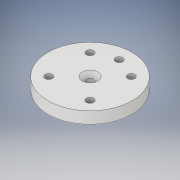
# Autodesk Inventor part: baseplate
Saved by Autodesk Inventor 2019 (Build 230136000, 136)
## iProperties
Created: 2019-05-05
Part Number: baseplate
Material: PBT Plastic
Document SubType Name: Modeling
Designer: infinity
Density: 1.31 g/cm^3
Appearance: Smooth - White
Author: infinity
Autodesk Inventor part; units mm, degrees
ref_plane "YZ Plane" through (0, 0, 0) normal (1, 0, 0) x (0, 1, 0)
ref_plane "XZ Plane" through (0, 0, 0) normal (0, 1, 0) x (-1, 0, 0)
ref_plane "XY Plane" through (0, 0, 0) normal (0, 0, 1) x (1, 0, 0)
sketch "Sketch1" plane through (0, 0, 0) normal (0, 1, 0) x (-1, 0, 0)
  circle A0 centre (0, 0) radius 36
  dimension "d0" = 72
  constraints: 1 centre point, 1 coincident
  measures "d0" diameter of A0
extrude "Extrusion1" add sketch "Sketch1" along normal blind 11
sketch "Sketch2" plane through (0, 0, 0) normal (0, -1, 0) x (1, 0, 0)
  line L0 (0, -58.3451) -> (0, 0) construction
  line L1 (0, 0) -> (-17.6777, -17.6777) construction
  point P0 (0, -25)
  point P1 (17.6777, -17.6777)
  point P2 (17.6777, 17.6777)
  point P3 (-17.6777, 17.6777)
  dimension "d84" = 45
  dimension "d85" = 25
  dimension "d86" = 25
  dimension "d89" = 360
  constraints: 4 end point, 1 point on line, 1 vertical, 5 other
  measures "d84" angle of L0 L1
  measures "d85" distance of L0.end L1.end
  measures "d86" distance of L0.end point (0, -25)
fillet "Fillet2" radius 1 1 edges at (36, 0, 0)
sketch "Sketch10" plane through (0, 0, 0) normal (0, -1, 0) x (1, 0, 0)
  circle A0 centre (0, 0) radius 15
  dimension "d66" = 30
  constraints: 1 centre point, 1 coincident
  measures "d66" diameter of A0
extrude "Extrusion6" add sketch "Sketch10" along normal blind 9
fillet "Fillet4" radius 3.175 1 edges at (-15, 0, 0)
sketch "Sketch11" plane through (0, -9, 0) normal (0, -1, 0) x (1, 0, 0)
  line L0 (-8.5, -4.2426) -> (-8.5, 4.2426)
  line L1 (8.5, 4.2426) -> (8.5, -4.2426)
  arc A0 (-8.5, -4.2426) -> (8.5, -4.2426) centre (0, 0) ccw
  arc A1 (8.5, 4.2426) -> (-8.5, 4.2426) centre (0, 0) ccw
  dimension "d71" = 17
  dimension "d72" = 8.5
  dimension "d73" = 9.5
  dimension "d74" = 9.5
  constraints: 4 end point, 4 point on circle, 2 centre point, 1 coincident, 1 parallel, 1 vertical
  measures "d71" distance between parallel lines of L1 L0
  measures "d72" distance from line of point (0, 0) L0
  measures "d73" radius of A1
  measures "d74" radius of A0
extrude "Extrusion7" cut sketch "Sketch11" against normal blind 9
sketch "Sketch12" plane through (0, 11, 0) normal (0, 1, 0) x (1, 0, 0)
  point P0 (0, 0)
  point P1 (0, 0)
  constraints: 1 coincident
hole "Hole5" at (0, 11, 0) direction (0, -1, 0) diameter 6.2 end through all countersink diameter 13.44 countersink angle 90
hole "Hole6" at (-17.6777, 0, -17.6777) at (0, 0, -25) at (17.6777, 0, -17.6777) at (17.6777, 0, 17.6777) at (-17.6777, 0, 17.6777) direction (0, 1, 0) diameter 6.2 end through all
equation "\"d72\" = 0.5 * d71"
body "Solid1"
